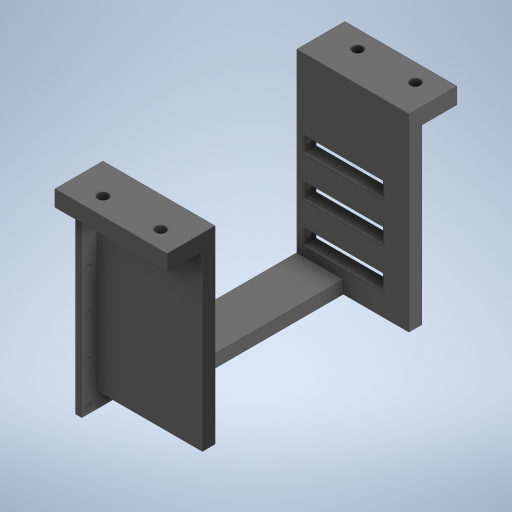
# Autodesk Inventor part: LeicTransfer Halter
Saved by Autodesk Inventor 2023 (Build 270158030, 158C)
## iProperties
Created: 2020-10-05
Part Number: LeicTransfer Halter
Material: Generic
Document SubType Name: Modeling
Designer: Julian
Density: 1 g/cm^3
Appearance: Default
Author: Julian
Autodesk Inventor part; units mm, degrees
ref_plane "YZ Plane" through (0, 0, 0) normal (1, 0, 0) x (0, 1, 0)
ref_plane "XZ Plane" through (0, 0, 0) normal (0, 1, 0) x (-1, 0, 0)
ref_plane "XY Plane" through (0, 0, 0) normal (0, 0, 1) x (1, 0, 0)
sketch "Sketch1" plane through (0, 0, 0) normal (1, 0, 0) x (0, 1, 0)
  line L0 (0, 0) -> (121, 0)
  line L1 (121, 0) -> (121, 121)
  line L2 (121, 121) -> (0, 121)
  line L3 (0, 121) -> (0, 0)
  line L4 (121, 0) -> (0, 0)
  line L5 (0, 0) -> (0, -8)
  line L6 (0, -8) -> (121, -8)
  line L7 (121, -8) -> (121, 0)
  line L8 (0, 121) -> (-14.1, 121)
  line L9 (-14.1, 121) -> (-14.1, 0)
  line L10 (-14.1, 0) -> (0, 0)
  line L11 (0, 0) -> (0, 121)
  line L12 (-14.1, 0) -> (0, 0)
  line L13 (0, 0) -> (0, -8)
  line L14 (0, -8) -> (-14.1, -8)
  line L15 (-14.1, -8) -> (-14.1, 0)
  line L16 (-14.1, 0) -> (-14.1, -3.25)
  line L17 (-14.1, -3.25) -> (10.9, -3.25)
  line L18 (10.9, -3.25) -> (35.9, -3.25)
  line L19 (35.9, -3.25) -> (60.9, -3.25)
  circle A0 centre (60.9, -3.25) radius 2.05
  circle A1 centre (35.9, -3.25) radius 2.05
  circle A2 centre (10.9, -3.25) radius 2.05
  circle A3 centre (-14.1, -3.25) radius 2.05
  line L20 (-14.1, -8) -> (-18.1, -8)
  line L21 (-18.1, -8) -> (-18.1, 121)
  line L22 (-18.1, 121) -> (-14.1, 121)
  line L23 (-14.1, 121) -> (-14.1, -8)
  line L24 (-18.1, 121) -> (120.9, 121)
  line L25 (120.9, 121) -> (120.9, 138.25)
  line L26 (120.9, 138.25) -> (-18.1, 138.25)
  line L27 (-18.1, 138.25) -> (-18.1, 121)
  line L28 (-14.1, -3.25) -> (-14.1, 21.75)
  line L29 (-14.1, 21.75) -> (-14.1, 46.75)
  line L30 (-14.1, 46.75) -> (-14.1, 71.75)
  line L31 (-14.1, 71.75) -> (-14.1, 96.75)
  line L32 (-14.1, 96.75) -> (-14.1, 121.75)
  line L33 (-14.1, 121.75) -> (-14.1, 134.25)
  line L34 (-14.1, 134.25) -> (10.9, 134.25)
  line L35 (10.9, 134.25) -> (35.9, 134.25)
  line L36 (35.9, 134.25) -> (60.9, 134.25)
  circle A4 centre (60.9, 134.25) radius 2.05
  circle A5 centre (35.9, 134.25) radius 2.05
  circle A6 centre (10.9, 134.25) radius 2.05
  circle A7 centre (-14.1, 134.25) radius 2.05
  circle A8 centre (-14.1, 121) radius 2.05
  circle A9 centre (-14.1, 96.75) radius 2.05
  circle A10 centre (-14.1, 71.75) radius 2.05
  circle A11 centre (-14.1, 46.75) radius 2.05
  circle A12 centre (-14.1, 21.75) radius 2.05
  line L37 (0, 121) -> (100, 121)
  line L38 (100, 121) -> (100, 129)
  line L39 (100, 129) -> (0, 129)
  line L40 (0, 129) -> (0, 121)
  line L41 (0, 129) -> (-8, 129)
  line L42 (-8, 129) -> (-8, -8)
  line L43 (-8, -8) -> (0, -8)
  line L44 (0, -8) -> (0, 129)
  line L45 (100, 129) -> (100, -8)
  line L46 (100, 129) -> (100, 138.25)
  line L47 (100, 121) -> (110, 121)
  line L48 (110, 121) -> (110, 151)
  line L49 (110, 151) -> (100, 151)
  line L50 (100, 151) -> (100, 121)
  line L51 (100, 0) -> (110, 0)
  line L52 (110, 0) -> (110, -30)
  line L53 (110, -30) -> (100, -30)
  line L54 (100, -30) -> (100, 0)
  point P0 (100, 0)
  point P1 (-8, 0)
  point P2 (-8, 121)
  point P3 (100, -8)
  dimension "d0" = 121
  dimension "d1" = 121
  dimension "d2" = 8
  dimension "d3" = 14.1
  dimension "d4" = 3.25
  dimension "d5" = 25
  dimension "d6" = 25
  dimension "d7" = 25
  dimension "d8" = 4.1
  dimension "d9" = 4.1
  dimension "d10" = 4.1
  dimension "d11" = 4.1
  dimension "d12" = 4
  dimension "d13" = 139
  dimension "d14" = 17.25
  dimension "d15" = 25
  dimension "d16" = 25
  dimension "d17" = 25
  dimension "d18" = 25
  dimension "d19" = 25
  dimension "d20" = 12.5
  dimension "d21" = 25
  dimension "d22" = 25
  dimension "d24" = 25
  dimension "d25" = 4.1
  dimension "d26" = 100
  dimension "d27" = 8
  dimension "d28" = 8
  dimension "d37" = 10
  dimension "d38" = 30
  dimension "d39" = 10
  dimension "d40" = 30
  constraints: 110 end point, 21 equal length, 16 point on line, 13 centre point, 13 coincident, 12 perpendicular, 11 horizontal, 1 vertical
  measures "d0" distance of L2.end L1.end
  measures "d1" distance of L1.end L0.end
  measures "d2" distance of L5.end L4.end
  measures "d3" distance of L10.end L9.end
  measures "d4" distance of L9.end L16.end
  measures "d5" distance of L16.end L17.end
  measures "d6" distance of L17.end L18.end
  measures "d7" distance of L18.end L19.end
  measures "d8" diameter of A0
  measures "d9" diameter of A1
  measures "d10" diameter of A2
  measures "d11" diameter of A3
  measures "d12" distance of L21.end L22.end
  measures "d13" distance of L26.end L25.end
  measures "d14" distance of L25.end L24.end
  measures "d15" distance of L28.start L28.end
  measures "d16" distance of L28.end L29.end
  measures "d17" distance of L29.end L30.end
  measures "d18" distance of L30.end L31.end
  measures "d19" distance of L31.end L32.end
  measures "d20" distance of L32.end L33.end
  measures "d21" distance of L33.end L34.end
  measures "d22" distance of L34.end L35.end
  measures "d24" distance of L35.end L36.end
  measures "d25" diameter of A8
  measures "d26" distance of L39.end L38.end
  measures "d27" distance of L38.end L37.end
  measures "d28" distance of L43.end L42.end
  measures "d37" distance of L49.end L48.end
  measures "d38" distance of L48.end L47.end
  measures "d39" distance of L52.end L53.end
  measures "d40" distance of L51.end L52.end
extrude "Extrusion2" add sketch "Sketch1" along normal blind 4 contours L42 L17 A3 L15 L10 | L10 L9 A12 A11 A10 A9 A8 L8 L42 | L8 A8 L22 L27 L26 L46 L39 L41 L42 | L42 L14 L15 A3 L17 | L15 A3 L20 L21 L22 A8 L9 A9 A10 A11 A12
extrude "Extrusion3" add sketch "Sketch1" along normal blind 70 contours L0 L45 L6 L5 | L5 L17 L42 L10 | L0 L52 L6 L45 | L40 L39 L38 L2 | L8 L42 L41 L40 | L5 L14 L42 L17 | L38 L46 L26 L48 L2 | L6 L52 L53 L54 | L26 L50 L49 L48 | A2 L18 L17 | L17 L18 A2 | A1 L19 L18 | L18 L19 A1 | A0
extrude "Extrusion4" add sketch "Sketch1" along normal blind 40 contours L10 L42 L8 L3
extrude "Extrusion5" cut sketch "Sketch1" along normal blind 4 contours A2 L18 L17 | L17 L18 A2 | A1 L19 L18 | L18 L19 A1 | A0
sketch "Sketch2" plane through (4, -18.1, -8) normal (0, 0, -1) x (-1, 0, 0)
  line L0 (0, 24) -> (-50, 24)
  line L1 (-50, 24) -> (-50, 34)
  line L2 (-50, 34) -> (0, 34)
  line L3 (0, 34) -> (0, 24)
  line L4 (4, 26.95) -> (4, 31.05) projected
  line L5 (4, 29) -> (0, 29)
  line L6 (0, 10.1) -> (0, 118.1) projected
  line L7 (0, 29) -> (0, 24)
  point P0 (4, 18.1)
  dimension "d43" = 50
  dimension "d44" = 10
  dimension "d45" = 5
  constraints: 12 end point, 2 horizontal, 2 parallel, 1 collinear, 1 midpoint, 1 perpendicular, 1 point on line
  measures "d43" distance of L1.end L2.end
  measures "d44" distance of L0.end L1.end
  measures "d45" distance between parallel lines of L5 L0
extrude "Extrusion6" cut sketch "Sketch2" against normal blind 10
pattern_linear "Rectangular Pattern1" count 3 spacing 25 along (0, 1, 0) of "Extrusion6"
sketch "Sketch3" plane through (0, 100, 138.25) normal (0, -1, 0) x (1, 0, 0)
  line L0 (0, 12.75) -> (70, 12.75) projected
  line L1 (70, 12.75) -> (55, 12.75)
  line L2 (55, 12.75) -> (55, 1.75)
  line L3 (55, 1.75) -> (70, 1.75)
  line L4 (70, 1.75) -> (70, 12.75)
  line L5 (55, 1.75) -> (19, 1.75)
  point P0 (0, -138.25)
  dimension "d51" = 15
  dimension "d52" = 11
  dimension "d53" = 36
  constraints: 10 end point, 2 horizontal, 2 parallel, 1 perpendicular
  measures "d51" distance of L3.end L2.end
  measures "d52" distance of L2.end L1.end
  measures "d53" distance of L2.end L5.end
hole "Hole1" at (55, 100, 140) at (19, 100, 140) direction (0, 1, 0) diameter 6.3 end through all counterbore diameter 12 counterbore depth 5 clearance for "Socket Head Cap Screw" size "M6" standard "Ansi Metric M Profile"
ref_plane "Work Plane1" through (70, 110, 60.5) normal (0, 0, -1) x (-1, 0, 0)
mirror "Mirror1" about plane through (70, 110, 60.5) normal (0, 0, -1) of "Hole1"
thicken "Thicken1" operation add thickness 11 both sides no extend neighbours yes toward (-1, 0, 0) faces at (40, -5.3333, 80.6667)
body "Solid1"
